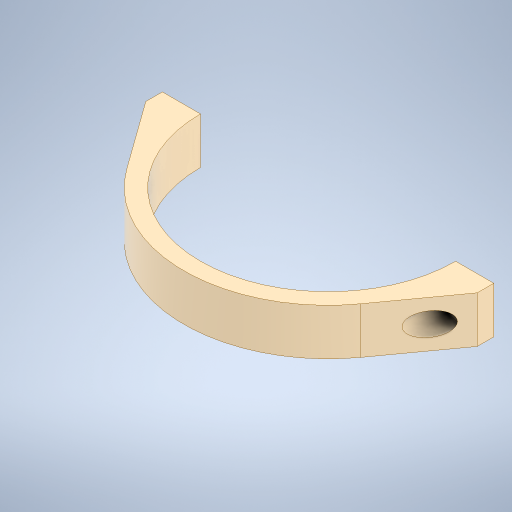
# Autodesk Inventor part: clamp
Saved by Autodesk Inventor 2024 (Build 280153020, 153B)
## iProperties
Created: 2023-06-12
Part Number: clamp
Material: Polyethylene, High Density
Document SubType Name: Modeling
Designer: OKESH
Density: 0.952 g/cm^3
Appearance: Smooth - Off-White
Author: OKESH
Autodesk Inventor part; units mm, degrees
ref_plane "YZ Plane" through (0, 0, 0) normal (1, 0, 0) x (0, 1, 0)
ref_plane "XZ Plane" through (0, 0, 0) normal (0, 1, 0) x (-1, 0, 0)
sketch "Sketch2" plane through (0, 0, 0) normal (0, 1, 0) x (-1, 0, 0)
  line L0 (-50, 0) -> (-50, 5)
  line L1 (50, 5) -> (50, 0)
  arc A0 (38.5, 0) -> (-38.5, 0) centre (0, 0) ccw
  line L2 (50, 5) -> (35.3035, 25.4148)
  line L3 (-50, 5) -> (-35.3035, 25.4148)
  line L4 (50, 0) -> (38.5, 0)
  line L5 (-38.5, 0) -> (-50, 0)
  line L6 (43.2117, 5) -> (50, 5)
  arc A1 (35.3035, 25.4148) -> (-35.3035, 25.4148) centre (0, 0) ccw
  point P0 (50, 2.5)
  dimension "d0" = 77
  dimension "d2" = 5
  dimension "d3" = 100
  dimension "d4" = 50
  constraints: 14 end point, 4 point on circle, 3 parallel, 2 centre point, 2 horizontal, 2 perpendicular, 2 tangent, 1 coincident, 1 midpoint
  measures "d0" diameter of A0
  measures "d2" distance of L1.start L1.end
  measures "d3" distance of L1.end L0.start
  measures "d4" horizontal distance of point (0, 0) point (50, 2.5)
extrude "Extrusion1" add sketch "Sketch2" along normal blind 14
ref_plane "Work Plane1" through (0, 0, 50) normal (0, 0, 1) x (1, 0, 0)
sketch "Sketch3" plane through (0, 0, 50) normal (0, 0, 1) x (1, 0, 0)
  line L0 (-38.5, 0) -> (-38.5, 14) projected
  circle A0 centre (44, 7) radius 2.5
  circle A1 centre (44, 7) radius 3.5
  line L1 (0, 0) -> (0, 17.8681)
  circle A2 centre (-44, 7) radius 2.5
  circle A3 centre (-44, 7) radius 3.5
  line L2 (35.3035, 14) -> (50, 14) projected
  dimension "d10" = 1
  dimension "d11" = 44
  dimension "d12" = 7
  constraints: 4 centre point, 2 end point, 1 symmetric about line, 1 vertical, 2 other
  measures "d10" radial gap between concentric circles of A0 A1
  measures "d11" horizontal distance of A0.centre L1.start
  measures "d12" distance from line of L2 A0.centre
extrude "Extrusion2" cut sketch "Sketch3" against normal blind 45
extrude "Extrusion3" cut sketch "Sketch3" against normal blind 60 contours A0 | A2
body "Solid1"
